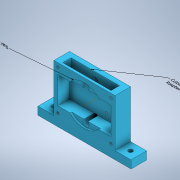
# Autodesk Inventor part: 2020PiZeroCameraLightRingMount
Saved by Autodesk Inventor 2020.2 (Build 242310000, 310)
## iProperties
Created: 2019-10-10
Part Number: 2020PiZeroCameraLightRingMount
Material: PC/ABS Plastic
Document SubType Name: Modeling
Designer: steele
Density: 0.357273 g/cm^3
Appearance: Turquoise
Author: steele
Autodesk Inventor part; units mm, degrees
ref_plane "YZ Plane" through (0, 0, 0) normal (1, 0, 0) x (0, 1, 0)
ref_plane "XZ Plane" through (0, 0, 0) normal (0, 1, 0) x (-1, 0, 0)
ref_plane "XY Plane" through (0, 0, 0) normal (0, 0, 1) x (1, 0, 0)
sketch "Sketch1" plane through (0, 0, 0) normal (0, 0, 1) x (1, 0, 0)
  line L0 (-48.5775, -37.85) -> (48.5775, -37.85)
  line L1 (48.5775, -37.85) -> (48.5775, 37.85)
  line L2 (48.5775, 37.85) -> (-48.5775, 37.85)
  line L3 (-48.5775, 37.85) -> (-48.5775, -37.85)
  line L4 (-48.5775, -37.85) -> (48.5775, 37.85) construction
  line L5 (48.5775, -37.85) -> (-48.5775, 37.85) construction
  point P0 (0, 0)
  dimension "majorPartWidth" = 97.155
  dimension "majorPartHeight" = 75.7
  constraints: 12 end point, 2 midpoint, 2 parallel, 1 horizontal, 1 perpendicular
  measures "majorPartWidth" distance of L0.start L0.end
  measures "majorPartHeight" distance of L1.end L0.end
extrude "Extrusion1" add sketch "Sketch1" against normal blind 24.725
sketch "Sketch2" plane through (0, 0, 0) normal (0, 0, 1) x (1, 0, 0)
  line L0 (-42.2275, -21.59) -> (42.2275, -21.59)
  line L1 (42.2275, -21.59) -> (42.2275, 21.59)
  line L2 (42.2275, 21.59) -> (-42.2275, 21.59)
  line L3 (-42.2275, 21.59) -> (-42.2275, -21.59)
  line L4 (-42.2275, -21.59) -> (42.2275, 21.59) construction
  line L5 (42.2275, -21.59) -> (-42.2275, 21.59) construction
  point P0 (0, 0)
  dimension "holeForPiCaseWidth" = 84.455
  dimension "holeForPiCaseHeight" = 43.18
  constraints: 12 end point, 2 midpoint, 2 parallel, 1 horizontal, 1 perpendicular
  measures "holeForPiCaseWidth" distance of L0.start L0.end
  measures "holeForPiCaseHeight" distance of L1.end L0.end
extrude "Extrusion2" cut sketch "Sketch2" against normal blind 18.375
sketch "Sketch3" plane through (0, 0, 0) normal (0, 0, 1) x (1, 0, 0)
  circle A0 centre (0, 0) radius 31.5
  circle A1 centre (0, 0) radius 18.5
  dimension "lightRingHoleExteriorDiam" = 63
  dimension "lightRingHoleInteriorDiam" = 37
  constraints: 2 centre point, 2 coincident
  measures "lightRingHoleExteriorDiam" diameter of A0
  measures "lightRingHoleInteriorDiam" diameter of A1
extrude "Extrusion3" cut sketch "Sketch3" against normal blind 2.5
sketch "Sketch4" plane through (0, 0, -2.5) normal (0, 0, 1) x (1, 0, 0)
  circle A0 centre (0, 0) radius 25.4466 construction
  circle A1 centre (0, 25.4466) radius 5
  circle A2 centre (0, -25.4466) radius 5
  dimension "holeForLightRingWires" = 10
  dimension "d13" = 10
  constraints: 3 centre point, 2 point on circle, 1 coincident
  measures "holeForLightRingWires" diameter of A1
  measures "d13" diameter of A2
extrude "Extrusion4" cut sketch "Sketch4" against normal through all
sketch "Sketch6" plane through (-48.5775, -37.85, 0) normal (0, -1, 0) x (1, 0, 0)
  line L0 (0, -24.725) -> (97.155, -24.725) projected
  line L1 (0, -24.725) -> (97.155, -24.725)
  line L2 (97.155, -24.725) -> (97.155, 0)
  line L3 (97.155, 0) -> (0, 0)
  line L4 (0, 0) -> (0, -24.725)
  point P0 (48.5775, 0)
  dimension "baseWidth" = 97.155
  dimension "baseDepth" = 24.725
  constraints: 8 end point, 2 parallel, 1 horizontal, 1 perpendicular
  measures "baseWidth" distance of L2.end L3.end
  measures "baseDepth" distance of L1.end L2.end
extrude "Extrusion6" add sketch "Sketch6" along normal blind 12.7
sketch "Sketch7" plane through (-48.5775, 37.85, 0) normal (0, 1, 0) x (1, 0, 0)
  line L0 (97.155, 0) -> (0, 0) construction
  line L1 (0, 0) -> (0, 24.725) construction
  line L2 (10.16, 3.77) -> (86.995, 3.77)
  line L3 (86.995, 3.77) -> (86.995, 17.105)
  line L4 (86.995, 17.105) -> (10.16, 17.105)
  line L5 (10.16, 17.105) -> (10.16, 3.77)
  line L6 (10.16, 3.77) -> (86.995, 17.105) construction
  line L7 (86.995, 3.77) -> (10.16, 17.105) construction
  line L8 (45.3952, 18.375) -> (45.3952, 2.5) projected
  point P0 (48.5775, 0)
  point P1 (48.5775, 10.4375)
  dimension "y" = 10.4375
  dimension "Y" = 48.5775
  dimension "piWireDepth" = 13.335
  dimension "piWireWidth" = 76.835
  constraints: 12 end point, 2 midpoint, 2 parallel, 2 perpendicular
  measures "y" distance from line of point (48.577, 10.438) L0
  measures "Y" distance from line of point (48.577, 10.438) L1
  measures "piWireDepth" distance of L4.end L2.start
  measures "piWireWidth" distance of L3.end L4.end
extrude "Extrusion7" cut sketch "Sketch7" against normal up to next
sketch "Sketch8" plane through (-48.5775, 37.85, -24.725) normal (-1, 0, 0) x (0, 0, 1)
  line L0 (24.725, -75.7) -> (24.725, 0) projected
  line L1 (24.725, -75.7) -> (28.535, -75.7)
  line L2 (28.535, -75.7) -> (28.535, -78.24)
  line L3 (28.535, -78.24) -> (24.725, -78.24)
  line L4 (24.725, -78.24) -> (24.725, -75.7)
  point P0 (24.725, -37.85)
  dimension "d30" = 3.81
  dimension "d31" = 2.54
  constraints: 8 end point, 2 parallel, 1 horizontal, 1 perpendicular
  measures "d30" distance of L2.end L3.end
  measures "d31" distance of L1.end L2.end
extrude "Extrusion8" cut sketch "Sketch8" against normal through all
sketch "Sketch9" plane through (0, 0, 0) normal (0, 0, 1) x (1, 0, 0)
  point P0 (-42.2275, 31.5)
  point P1 (42.2275, 31.5)
  point P2 (42.2275, -31.5)
  point P3 (-42.2275, -31.5)
hole "Hole1" at (-42.2275, 31.5, 0) at (42.2275, 31.5, 0) at (42.2275, -31.5, 0) at (-42.2275, -31.5, 0) direction (0, 0, -1) diameter 3.9624 depth 14.986 tip angle 120 thread size "10-32 UNF" class "2B" standard "ANSI Unified Screw Threads"
sketch "Sketch10" plane through (0, 0, -24.725) normal (0, 0, -1) x (-1, 0, 0)
  point P0 (-39.0525, 23.7022)
  point P1 (-16.8275, 23.7022)
  point P2 (-16.8275, -11.2228)
  point P3 (-39.0525, -11.2228)
hole "Hole3" at (39.0525, 23.7022, -24.725) at (16.8275, 23.7022, -24.725) at (16.8275, -11.2228, -24.725) at (39.0525, -11.2228, -24.725) direction (0, 0, 1) diameter 3.9624 depth 11.9507 tip angle 120 thread size "10-32 UNF" class "2B" standard "ANSI Unified Screw Threads"
sketch "Sketch14" plane through (-48.5775, -50.55, 0) normal (0, -1, 0) x (1, 0, 0)
  circle A0 centre (-12.7, 0) radius 2.5527 construction
  circle A1 centre (109.855, 0) radius 2.5527 construction
  line L0 (-12.7, 0) -> (109.855, 0) construction
  spline S0 degree 2 poles (41.3517, -2.5421) (41.3517, -2.8899) (41.0697, -3.4498) (40.833, -3.6062) knots 0 0 0 1 2 2 2
  spline S1 degree 2 poles (40.833, -3.6062) (40.6395, -3.7277) (40.2422, -3.81) (39.9335, -3.81) knots 0 0 0 1 2 2 2
  line L1 (39.9335, -3.81) -> (39.3489, -3.81)
  line L2 (39.3489, -3.81) -> (39.3489, -1.27)
  line L3 (39.3489, -1.27) -> (39.9273, -1.27)
  spline S2 degree 2 poles (39.9273, -1.27) (40.2854, -1.27) (40.693, -1.377) (40.8371, -1.4717) knots 0 0 0 1 2 2 2
  spline S3 degree 2 poles (40.8371, -1.4717) (41.082, -1.6343) (41.3517, -2.1716) (41.3517, -2.5421) knots 0 0 0 1 2 2 2
  spline S4 degree 2 poles (40.9997, -2.5379) (40.9997, -2.2457) (40.8062, -1.8319) (40.6148, -1.7146) knots 0 0 0 1 2 2 2
  spline S5 degree 2 poles (40.6148, -1.7146) (40.4789, -1.6343) (40.1722, -1.5623) (39.9438, -1.5623) knots 0 0 0 1 2 2 2
  line L4 (39.9438, -1.5623) -> (39.6865, -1.5623)
  line L5 (39.6865, -1.5623) -> (39.6865, -3.5177)
  line L6 (39.6865, -3.5177) -> (39.9438, -3.5177)
  spline S6 degree 2 poles (39.9438, -3.5177) (40.1681, -3.5177) (40.5078, -3.4457) (40.6457, -3.3489) knots 0 0 0 1 2 2 2
  spline S7 degree 2 poles (40.6457, -3.3489) (40.8227, -3.2295) (40.9997, -2.8343) (40.9997, -2.5379) knots 0 0 0 1 2 2 2
  spline S8 degree 2 poles (42.5208, -3.8532) (42.0639, -3.8532) (41.5616, -3.3407) (41.5616, -2.8673) knots 0 0 0 1 2 2 2
  spline S9 degree 2 poles (41.5616, -2.8673) (41.5616, -2.4021) (42.0495, -1.8505) (42.4426, -1.8505) knots 0 0 0 1 2 2 2
  spline S10 degree 2 poles (42.4426, -1.8505) (42.6196, -1.8505) (42.8934, -1.9534) (42.9942, -2.0625) knots 0 0 0 1 2 2 2
  spline S11 degree 2 poles (42.9942, -2.0625) (43.0972, -2.1716) (43.2062, -2.4865) (43.2062, -2.715) knots 0 0 0 1 2 2 2
  line L7 (43.2062, -2.715) -> (43.2062, -2.8899)
  line L8 (43.2062, -2.8899) -> (41.8868, -2.8899)
  spline S12 degree 2 poles (41.8868, -2.8899) (41.8868, -3.2213) (42.2203, -3.5733) (42.5167, -3.5733) knots 0 0 0 1 2 2 2
  spline S13 degree 2 poles (42.5167, -3.5733) (42.6217, -3.5733) (42.8254, -3.5259) (42.9078, -3.4889) knots 0 0 0 1 2 2 2
  spline S14 degree 2 poles (42.9078, -3.4889) (42.9942, -3.4477) (43.1136, -3.3757) (43.1527, -3.3428) knots 0 0 0 1 2 2 2
  line L9 (43.1527, -3.3428) -> (43.1713, -3.3428)
  line L10 (43.1713, -3.3428) -> (43.1713, -3.6927)
  spline S15 degree 2 poles (43.1713, -3.6927) (43.1157, -3.7153) (42.9469, -3.7812) (42.881, -3.7997) knots 0 0 0 1 2 2 2
  spline S16 degree 2 poles (42.881, -3.7997) (42.7884, -3.8265) (42.6361, -3.8532) (42.5208, -3.8532) knots 0 0 0 1 2 2 2
  spline S17 degree 2 poles (42.8934, -2.645) (42.8893, -2.5153) (42.8357, -2.3259) (42.7843, -2.2621) knots 0 0 0 1 2 2 2
  spline S18 degree 2 poles (42.7843, -2.2621) (42.7287, -2.1901) (42.5537, -2.1139) (42.4241, -2.1139) knots 0 0 0 1 2 2 2
  spline S19 degree 2 poles (42.4241, -2.1139) (42.2965, -2.1139) (42.1174, -2.1901) (42.0433, -2.2642) knots 0 0 0 1 2 2 2
  spline S20 degree 2 poles (42.0433, -2.2642) (41.9712, -2.3403) (41.8971, -2.5235) (41.8868, -2.645) knots 0 0 0 1 2 2 2
  line L11 (41.8868, -2.645) -> (42.8934, -2.645)
  spline S21 degree 2 poles (44.046, -3.8553) (43.8546, -3.8553) (43.5232, -3.7524) (43.4141, -3.6947) knots 0 0 0 1 2 2 2
  line L12 (43.4141, -3.6947) -> (43.4141, -3.3345)
  line L13 (43.4141, -3.3345) -> (43.4306, -3.3345)
  spline S22 degree 2 poles (43.4306, -3.3345) (43.4718, -3.3675) (43.5829, -3.4457) (43.6755, -3.4889) knots 0 0 0 1 2 2 2
  spline S23 degree 2 poles (43.6755, -3.4889) (43.7558, -3.528) (43.9534, -3.5856) (44.0584, -3.5856) knots 0 0 0 1 2 2 2
  spline S24 degree 2 poles (44.0584, -3.5856) (44.1346, -3.5856) (44.3095, -3.5506) (44.3507, -3.5218) knots 0 0 0 1 2 2 2
  spline S25 degree 2 poles (44.3507, -3.5218) (44.4104, -3.4827) (44.4639, -3.3942) (44.4639, -3.3036) knots 0 0 0 1 2 2 2
  spline S26 degree 2 poles (44.4639, -3.3036) (44.4639, -3.1904) (44.3404, -3.0731) (44.1819, -3.034) knots 0 0 0 1 2 2 2
  spline S27 degree 2 poles (44.1819, -3.034) (44.1202, -3.0196) (43.9225, -2.9784) (43.8382, -2.9558) knots 0 0 0 1 2 2 2
  spline S28 degree 2 poles (43.8382, -2.9558) (43.62, -2.892) (43.4224, -2.6285) (43.4224, -2.4412) knots 0 0 0 1 2 2 2
  spline S29 degree 2 poles (43.4224, -2.4412) (43.4224, -2.1818) (43.8114, -1.8587) (44.1325, -1.8587) knots 0 0 0 1 2 2 2
  spline S30 degree 2 poles (44.1325, -1.8587) (44.291, -1.8587) (44.6121, -1.9369) (44.7212, -1.9966) knots 0 0 0 1 2 2 2
  line L14 (44.7212, -1.9966) -> (44.7212, -2.3403)
  line L15 (44.7212, -2.3403) -> (44.7047, -2.3403)
  spline S31 degree 2 poles (44.7047, -2.3403) (44.5812, -2.2415) (44.2807, -2.1283) (44.1263, -2.1283) knots 0 0 0 1 2 2 2
  spline S32 degree 2 poles (44.1263, -2.1283) (43.9678, -2.1283) (43.7496, -2.2621) (43.7496, -2.3959) knots 0 0 0 1 2 2 2
  spline S33 degree 2 poles (43.7496, -2.3959) (43.7496, -2.5174) (43.8793, -2.6347) (44.0234, -2.6717) knots 0 0 0 1 2 2 2
  spline S34 degree 2 poles (44.0234, -2.6717) (44.0934, -2.6903) (44.2704, -2.7273) (44.3672, -2.75) knots 0 0 0 1 2 2 2
  spline S35 degree 2 poles (44.3672, -2.75) (44.5771, -2.8035) (44.7912, -3.0484) (44.7912, -3.2604) knots 0 0 0 1 2 2 2
  spline S36 degree 2 poles (44.7912, -3.2604) (44.7912, -3.3839) (44.6944, -3.6021) (44.5997, -3.6824) knots 0 0 0 1 2 2 2
  spline S37 degree 2 poles (44.5997, -3.6824) (44.4989, -3.7668) (44.2416, -3.8553) (44.046, -3.8553) knots 0 0 0 1 2 2 2
  line L16 (45.4169, -3.81) -> (45.0958, -3.81)
  line L17 (45.0958, -3.81) -> (45.0958, -1.904)
  line L18 (45.0958, -1.904) -> (45.4169, -1.904)
  line L19 (45.4169, -1.904) -> (45.4169, -3.81)
  line L20 (45.4396, -1.587) -> (45.0752, -1.587)
  line L21 (45.0752, -1.587) -> (45.0752, -1.2535)
  line L22 (45.0752, -1.2535) -> (45.4396, -1.2535)
  line L23 (45.4396, -1.2535) -> (45.4396, -1.587)
  spline S38 degree 2 poles (45.9562, -4.1146) (45.9891, -4.129) (46.1147, -4.1743) (46.195, -4.1929) knots 0 0 0 1 2 2 2
  spline S39 degree 2 poles (46.195, -4.1929) (46.2835, -4.2155) (46.4337, -4.2423) (46.5222, -4.2423) knots 0 0 0 1 2 2 2
  spline S40 degree 2 poles (46.5222, -4.2423) (46.6704, -4.2423) (46.8763, -4.164) (46.9339, -4.0941) knots 0 0 0 1 2 2 2
  spline S41 degree 2 poles (46.9339, -4.0941) (46.9895, -4.0241) (47.0327, -3.8409) (47.0327, -3.7235) knots 0 0 0 1 2 2 2
  line L24 (47.0327, -3.7235) -> (47.0327, -3.5568)
  spline S42 degree 2 poles (47.0327, -3.5568) (46.903, -3.67) (46.654, -3.7771) (46.4667, -3.7771) knots 0 0 0 1 2 2 2
  spline S43 degree 2 poles (46.4667, -3.7771) (46.1414, -3.7771) (45.7565, -3.2934) (45.7565, -2.8385) knots 0 0 0 1 2 2 2
  spline S44 degree 2 poles (45.7565, -2.8385) (45.7565, -2.6018) (45.8903, -2.2354) (46.0015, -2.1057) knots 0 0 0 1 2 2 2
  spline S45 degree 2 poles (46.0015, -2.1057) (46.1085, -1.9842) (46.4029, -1.8505) (46.5593, -1.8505) knots 0 0 0 1 2 2 2
  spline S46 degree 2 poles (46.5593, -1.8505) (46.7075, -1.8505) (46.9236, -1.9204) (47.0327, -1.9842) knots 0 0 0 1 2 2 2
  line L25 (47.0327, -1.9842) -> (47.0512, -1.904)
  line L26 (47.0512, -1.904) -> (47.3538, -1.904)
  line L27 (47.3538, -1.904) -> (47.3538, -3.5918)
  spline S47 degree 2 poles (47.3538, -3.5918) (47.3538, -4.0776) (46.9319, -4.5304) (46.4975, -4.5304) knots 0 0 0 1 2 2 2
  spline S48 degree 2 poles (46.4975, -4.5304) (46.3576, -4.5304) (46.0653, -4.4851) (45.9397, -4.4481) knots 0 0 0 1 2 2 2
  line L28 (45.9397, -4.4481) -> (45.9397, -4.1146)
  line L29 (45.9397, -4.1146) -> (45.9562, -4.1146)
  line L30 (47.0327, -3.2934) -> (47.0327, -2.2457)
  spline S49 degree 2 poles (47.0327, -2.2457) (46.9133, -2.188) (46.7116, -2.1386) (46.6107, -2.1386) knots 0 0 0 1 2 2 2
  spline S50 degree 2 poles (46.6107, -2.1386) (46.3679, -2.1386) (46.0879, -2.4968) (46.0879, -2.8323) knots 0 0 0 1 2 2 2
  spline S51 degree 2 poles (46.0879, -2.8323) (46.0879, -3.1493) (46.2999, -3.4807) (46.5387, -3.4807) knots 0 0 0 1 2 2 2
  spline S52 degree 2 poles (46.5387, -3.4807) (46.6643, -3.4807) (46.9277, -3.3819) (47.0327, -3.2934) knots 0 0 0 1 2 2 2
  line L31 (49.3154, -3.81) -> (48.9943, -3.81)
  line L32 (48.9943, -3.81) -> (48.9943, -2.7232)
  spline S53 degree 2 poles (48.9943, -2.7232) (48.9943, -2.5915) (48.9696, -2.365) (48.9326, -2.2971) knots 0 0 0 1 2 2 2
  spline S54 degree 2 poles (48.9326, -2.2971) (48.8935, -2.2251) (48.7535, -2.1551) (48.6341, -2.1551) knots 0 0 0 1 2 2 2
  spline S55 degree 2 poles (48.6341, -2.1551) (48.5147, -2.1551) (48.2615, -2.2827) (48.1401, -2.3856) knots 0 0 0 1 2 2 2
  line L33 (48.1401, -2.3856) -> (48.1401, -3.81)
  line L34 (48.1401, -3.81) -> (47.819, -3.81)
  line L35 (47.819, -3.81) -> (47.819, -1.904)
  line L36 (47.819, -1.904) -> (48.1401, -1.904)
  line L37 (48.1401, -1.904) -> (48.1401, -2.116)
  spline S56 degree 2 poles (48.1401, -2.116) (48.2842, -1.9863) (48.5621, -1.8505) (48.7185, -1.8505) knots 0 0 0 1 2 2 2
  spline S57 degree 2 poles (48.7185, -1.8505) (48.9984, -1.8505) (49.3154, -2.221) (49.3154, -2.5729) knots 0 0 0 1 2 2 2
  line L38 (49.3154, -2.5729) -> (49.3154, -3.81)
  spline S58 degree 2 poles (50.5937, -3.8532) (50.1367, -3.8532) (49.6345, -3.3407) (49.6345, -2.8673) knots 0 0 0 1 2 2 2
  spline S59 degree 2 poles (49.6345, -2.8673) (49.6345, -2.4021) (50.1223, -1.8505) (50.5154, -1.8505) knots 0 0 0 1 2 2 2
  spline S60 degree 2 poles (50.5154, -1.8505) (50.6925, -1.8505) (50.9662, -1.9534) (51.0671, -2.0625) knots 0 0 0 1 2 2 2
  spline S61 degree 2 poles (51.0671, -2.0625) (51.17, -2.1716) (51.2791, -2.4865) (51.2791, -2.715) knots 0 0 0 1 2 2 2
  line L39 (51.2791, -2.715) -> (51.2791, -2.8899)
  line L40 (51.2791, -2.8899) -> (49.9597, -2.8899)
  spline S62 degree 2 poles (49.9597, -2.8899) (49.9597, -3.2213) (50.2931, -3.5733) (50.5895, -3.5733) knots 0 0 0 1 2 2 2
  spline S63 degree 2 poles (50.5895, -3.5733) (50.6945, -3.5733) (50.8983, -3.5259) (50.9806, -3.4889) knots 0 0 0 1 2 2 2
  spline S64 degree 2 poles (50.9806, -3.4889) (51.0671, -3.4477) (51.1865, -3.3757) (51.2256, -3.3428) knots 0 0 0 1 2 2 2
  line L41 (51.2256, -3.3428) -> (51.2441, -3.3428)
  line L42 (51.2441, -3.3428) -> (51.2441, -3.6927)
  spline S65 degree 2 poles (51.2441, -3.6927) (51.1885, -3.7153) (51.0197, -3.7812) (50.9539, -3.7997) knots 0 0 0 1 2 2 2
  spline S66 degree 2 poles (50.9539, -3.7997) (50.8612, -3.8265) (50.7089, -3.8532) (50.5937, -3.8532) knots 0 0 0 1 2 2 2
  spline S67 degree 2 poles (50.9662, -2.645) (50.9621, -2.5153) (50.9086, -2.3259) (50.8571, -2.2621) knots 0 0 0 1 2 2 2
  spline S68 degree 2 poles (50.8571, -2.2621) (50.8015, -2.1901) (50.6266, -2.1139) (50.4969, -2.1139) knots 0 0 0 1 2 2 2
  spline S69 degree 2 poles (50.4969, -2.1139) (50.3693, -2.1139) (50.1902, -2.1901) (50.1161, -2.2642) knots 0 0 0 1 2 2 2
  spline S70 degree 2 poles (50.1161, -2.2642) (50.0441, -2.3403) (49.97, -2.5235) (49.9597, -2.645) knots 0 0 0 1 2 2 2
  line L43 (49.9597, -2.645) -> (50.9662, -2.645)
  line L44 (53.0698, -3.81) -> (52.7487, -3.81)
  line L45 (52.7487, -3.81) -> (52.7487, -3.6165)
  spline S71 degree 2 poles (52.7487, -3.6165) (52.6746, -3.6783) (52.5655, -3.7606) (52.4914, -3.7956) knots 0 0 0 1 2 2 2
  spline S72 degree 2 poles (52.4914, -3.7956) (52.4235, -3.8285) (52.2774, -3.8635) (52.1806, -3.8635) knots 0 0 0 1 2 2 2
  spline S73 degree 2 poles (52.1806, -3.8635) (52.0242, -3.8635) (51.7607, -3.7338) (51.6681, -3.6083) knots 0 0 0 1 2 2 2
  spline S74 degree 2 poles (51.6681, -3.6083) (51.5755, -3.4827) (51.4726, -3.1122) (51.4726, -2.8714) knots 0 0 0 1 2 2 2
  spline S75 degree 2 poles (51.4726, -2.8714) (51.4726, -2.6203) (51.6022, -2.2539) (51.7154, -2.116) knots 0 0 0 1 2 2 2
  spline S76 degree 2 poles (51.7154, -2.116) (51.8204, -1.9925) (52.1148, -1.8505) (52.2774, -1.8505) knots 0 0 0 1 2 2 2
  spline S77 degree 2 poles (52.2774, -1.8505) (52.4194, -1.8505) (52.6314, -1.9143) (52.7487, -1.9801) knots 0 0 0 1 2 2 2
  line L46 (52.7487, -1.9801) -> (52.7487, -1.1568)
  line L47 (52.7487, -1.1568) -> (53.0698, -1.1568)
  line L48 (53.0698, -1.1568) -> (53.0698, -3.81)
  line L49 (52.7487, -3.3469) -> (52.7487, -2.2457)
  spline S78 degree 2 poles (52.7487, -2.2457) (52.6294, -2.188) (52.44, -2.1448) (52.3309, -2.1448) knots 0 0 0 1 2 2 2
  spline S79 degree 2 poles (52.3309, -2.1448) (52.0839, -2.1448) (51.804, -2.5153) (51.804, -2.8652) knots 0 0 0 1 2 2 2
  spline S80 degree 2 poles (51.804, -2.8652) (51.804, -3.2028) (52.018, -3.5589) (52.2547, -3.5589) knots 0 0 0 1 2 2 2
  spline S81 degree 2 poles (52.2547, -3.5589) (52.3803, -3.5589) (52.6355, -3.4436) (52.7487, -3.3469) knots 0 0 0 1 2 2 2
  spline S82 degree 2 poles (56.2232, -2.8261) (56.2232, -3.2934) (55.7704, -3.8635) (55.4287, -3.8635) knots 0 0 0 1 2 2 2
  spline S83 degree 2 poles (55.4287, -3.8635) (55.2743, -3.8635) (55.0541, -3.7874) (54.9471, -3.7215) knots 0 0 0 1 2 2 2
  line L50 (54.9471, -3.7215) -> (54.9265, -3.81)
  line L51 (54.9265, -3.81) -> (54.626, -3.81)
  line L52 (54.626, -3.81) -> (54.626, -1.1568)
  line L53 (54.626, -1.1568) -> (54.9471, -1.1568)
  line L54 (54.9471, -1.1568) -> (54.9471, -2.1036)
  spline S84 degree 2 poles (54.9471, -2.1036) (55.0685, -1.9945) (55.3505, -1.8505) (55.5296, -1.8505) knots 0 0 0 1 2 2 2
  spline S85 degree 2 poles (55.5296, -1.8505) (55.8527, -1.8505) (56.2232, -2.3671) (56.2232, -2.8261) knots 0 0 0 1 2 2 2
  spline S86 degree 2 poles (55.8918, -2.8508) (55.8918, -2.5091) (55.6839, -2.1551) (55.4534, -2.1551) knots 0 0 0 1 2 2 2
  spline S87 degree 2 poles (55.4534, -2.1551) (55.3237, -2.1551) (55.0561, -2.2786) (54.9471, -2.3733) knots 0 0 0 1 2 2 2
  line L55 (54.9471, -2.3733) -> (54.9471, -3.4663)
  spline S88 degree 2 poles (54.9471, -3.4663) (55.0685, -3.5259) (55.2558, -3.5753) (55.367, -3.5753) knots 0 0 0 1 2 2 2
  spline S89 degree 2 poles (55.367, -3.5753) (55.6119, -3.5753) (55.8918, -3.2275) (55.8918, -2.8508) knots 0 0 0 1 2 2 2
  line L56 (58.0531, -1.904) -> (57.028, -4.5119)
  line L57 (57.028, -4.5119) -> (56.6843, -4.5119)
  line L58 (56.6843, -4.5119) -> (57.026, -3.7174)
  line L59 (57.026, -3.7174) -> (56.3344, -1.904)
  line L60 (56.3344, -1.904) -> (56.6802, -1.904)
  line L61 (56.6802, -1.904) -> (57.2009, -3.316)
  line L62 (57.2009, -3.316) -> (57.7196, -1.904)
  line L63 (57.7196, -1.904) -> (58.0531, -1.904)
  line L64 (42.5445, -8.0641) -> (42.1061, -8.0641)
  line L65 (42.1061, -8.0641) -> (41.3033, -7.0535)
  line L66 (41.3033, -7.0535) -> (40.9163, -7.0535)
  line L67 (40.9163, -7.0535) -> (40.9163, -8.0641)
  line L68 (40.9163, -8.0641) -> (40.5788, -8.0641)
  line L69 (40.5788, -8.0641) -> (40.5788, -5.5241)
  line L70 (40.5788, -5.5241) -> (41.2333, -5.5241)
  spline S90 degree 2 poles (41.2333, -5.5241) (41.4515, -5.5241) (41.7458, -5.5715) (41.8796, -5.6579) knots 0 0 0 1 2 2 2
  spline S91 degree 2 poles (41.8796, -5.6579) (42.0134, -5.7444) (42.1678, -6.014) (42.1678, -6.2137) knots 0 0 0 1 2 2 2
  spline S92 degree 2 poles (42.1678, -6.2137) (42.1678, -6.4916) (41.8838, -6.8682) (41.6409, -6.9588) knots 0 0 0 1 2 2 2
  line L71 (41.6409, -6.9588) -> (42.5445, -8.0641)
  spline S93 degree 2 poles (41.8158, -6.2404) (41.8158, -6.1293) (41.7376, -5.9585) (41.6553, -5.9029) knots 0 0 0 1 2 2 2
  spline S94 degree 2 poles (41.6553, -5.9029) (41.5832, -5.8555) (41.3918, -5.8164) (41.2518, -5.8164) knots 0 0 0 1 2 2 2
  line L72 (41.2518, -5.8164) -> (40.9163, -5.8164)
  line L73 (40.9163, -5.8164) -> (40.9163, -6.7715)
  line L74 (40.9163, -6.7715) -> (41.2127, -6.7715)
  spline S95 degree 2 poles (41.2127, -6.7715) (41.3589, -6.7715) (41.5915, -6.72) (41.6717, -6.6398) knots 0 0 0 1 2 2 2
  spline S96 degree 2 poles (41.6717, -6.6398) (41.7458, -6.5698) (41.8158, -6.3722) (41.8158, -6.2404) knots 0 0 0 1 2 2 2
  spline S97 degree 2 poles (44.2879, -7.1111) (44.2879, -7.5928) (43.8248, -8.1177) (43.4378, -8.1177) knots 0 0 0 1 2 2 2
  spline S98 degree 2 poles (43.4378, -8.1177) (43.0405, -8.1177) (42.5857, -7.5763) (42.5857, -7.1111) knots 0 0 0 1 2 2 2
  spline S99 degree 2 poles (42.5857, -7.1111) (42.5857, -6.6336) (43.055, -6.1046) (43.4378, -6.1046) knots 0 0 0 1 2 2 2
  spline S100 degree 2 poles (43.4378, -6.1046) (43.8248, -6.1046) (44.2879, -6.6315) (44.2879, -7.1111) knots 0 0 0 1 2 2 2
  spline S101 degree 2 poles (43.9565, -7.1111) (43.9565, -6.7406) (43.6869, -6.3804) (43.4378, -6.3804) knots 0 0 0 1 2 2 2
  spline S102 degree 2 poles (43.4378, -6.3804) (43.1887, -6.3804) (42.917, -6.7406) (42.917, -7.1111) knots 0 0 0 1 2 2 2
  spline S103 degree 2 poles (42.917, -7.1111) (42.917, -7.4713) (43.1887, -7.8418) (43.4378, -7.8418) knots 0 0 0 1 2 2 2
  spline S104 degree 2 poles (43.4378, -7.8418) (43.6848, -7.8418) (43.9565, -7.4775) (43.9565, -7.1111) knots 0 0 0 1 2 2 2
  spline S105 degree 2 poles (46.2145, -7.0803) (46.2145, -7.5475) (45.7617, -8.1177) (45.42, -8.1177) knots 0 0 0 1 2 2 2
  spline S106 degree 2 poles (45.42, -8.1177) (45.2656, -8.1177) (45.0454, -8.0415) (44.9383, -7.9756) knots 0 0 0 1 2 2 2
  line L75 (44.9383, -7.9756) -> (44.9178, -8.0641)
  line L76 (44.9178, -8.0641) -> (44.6172, -8.0641)
  line L77 (44.6172, -8.0641) -> (44.6172, -5.4109)
  line L78 (44.6172, -5.4109) -> (44.9383, -5.4109)
  line L79 (44.9383, -5.4109) -> (44.9383, -6.3578)
  spline S107 degree 2 poles (44.9383, -6.3578) (45.0598, -6.2487) (45.3418, -6.1046) (45.5209, -6.1046) knots 0 0 0 1 2 2 2
  spline S108 degree 2 poles (45.5209, -6.1046) (45.844, -6.1046) (46.2145, -6.6212) (46.2145, -7.0803) knots 0 0 0 1 2 2 2
  spline S109 degree 2 poles (45.8831, -7.105) (45.8831, -6.7633) (45.6752, -6.4092) (45.4447, -6.4092) knots 0 0 0 1 2 2 2
  spline S110 degree 2 poles (45.4447, -6.4092) (45.315, -6.4092) (45.0474, -6.5327) (44.9383, -6.6274) knots 0 0 0 1 2 2 2
  line L80 (44.9383, -6.6274) -> (44.9383, -7.7204)
  spline S111 degree 2 poles (44.9383, -7.7204) (45.0598, -7.7801) (45.2471, -7.8295) (45.3582, -7.8295) knots 0 0 0 1 2 2 2
  spline S112 degree 2 poles (45.3582, -7.8295) (45.6032, -7.8295) (45.8831, -7.4816) (45.8831, -7.105) knots 0 0 0 1 2 2 2
  spline S113 degree 2 poles (48.3717, -8.1094) (48.0958, -8.1094) (47.7089, -7.9942) (47.538, -7.9118) knots 0 0 0 1 2 2 2
  line L81 (47.538, -7.9118) -> (47.538, -7.4878)
  line L82 (47.538, -7.4878) -> (47.5627, -7.4878)
  spline S114 degree 2 poles (47.5627, -7.4878) (47.7295, -7.6442) (48.1514, -7.8171) (48.347, -7.8171) knots 0 0 0 1 2 2 2
  spline S115 degree 2 poles (48.347, -7.8171) (48.6269, -7.8171) (48.913, -7.5845) (48.913, -7.3931) knots 0 0 0 1 2 2 2
  spline S116 degree 2 poles (48.913, -7.3931) (48.913, -7.2408) (48.7628, -7.0514) (48.6001, -7.0041) knots 0 0 0 1 2 2 2
  spline S117 degree 2 poles (48.6001, -7.0041) (48.4828, -6.9712) (48.2873, -6.9259) (48.1411, -6.8888) knots 0 0 0 1 2 2 2
  spline S118 degree 2 poles (48.1411, -6.8888) (48.0094, -6.8538) (47.8015, -6.7489) (47.7212, -6.6645) knots 0 0 0 1 2 2 2
  spline S119 degree 2 poles (47.7212, -6.6645) (47.643, -6.5801) (47.5566, -6.3537) (47.5566, -6.2055) knots 0 0 0 1 2 2 2
  spline S120 degree 2 poles (47.5566, -6.2055) (47.5566, -5.8967) (48.0382, -5.4789) (48.4108, -5.4789) knots 0 0 0 1 2 2 2
  spline S121 degree 2 poles (48.4108, -5.4789) (48.6248, -5.4789) (49.0036, -5.5633) (49.1662, -5.6435) knots 0 0 0 1 2 2 2
  line L83 (49.1662, -5.6435) -> (49.1662, -6.047)
  line L84 (49.1662, -6.047) -> (49.1415, -6.047)
  spline S122 degree 2 poles (49.1415, -6.047) (49.02, -5.9358) (48.6413, -5.7711) (48.4334, -5.7711) knots 0 0 0 1 2 2 2
  spline S123 degree 2 poles (48.4334, -5.7711) (48.1988, -5.7711) (47.9085, -5.9914) (47.9085, -6.1705) knots 0 0 0 1 2 2 2
  spline S124 degree 2 poles (47.9085, -6.1705) (47.9085, -6.331) (48.0794, -6.5224) (48.2399, -6.5657) knots 0 0 0 1 2 2 2
  spline S125 degree 2 poles (48.2399, -6.5657) (48.347, -6.5945) (48.6578, -6.6686) (48.7607, -6.6995) knots 0 0 0 1 2 2 2
  spline S126 degree 2 poles (48.7607, -6.6995) (49.0221, -6.7797) (49.265, -7.1029) (49.265, -7.3396) knots 0 0 0 1 2 2 2
  spline S127 degree 2 poles (49.265, -7.3396) (49.265, -7.4899) (49.1435, -7.778) (49.0345, -7.8789) knots 0 0 0 1 2 2 2
  spline S128 degree 2 poles (49.0345, -7.8789) (48.913, -7.99) (48.6043, -8.1094) (48.3717, -8.1094) knots 0 0 0 1 2 2 2
  spline S129 degree 2 poles (50.1604, -8.1012) (49.899, -8.1012) (49.6046, -7.8027) (49.6046, -7.4796) knots 0 0 0 1 2 2 2
  line L85 (49.6046, -7.4796) -> (49.6046, -6.4236)
  line L86 (49.6046, -6.4236) -> (49.3885, -6.4236)
  line L87 (49.3885, -6.4236) -> (49.3885, -6.1581)
  line L88 (49.3885, -6.1581) -> (49.6046, -6.1581)
  line L89 (49.6046, -6.1581) -> (49.6046, -5.6106)
  line L90 (49.6046, -5.6106) -> (49.9257, -5.6106)
  line L91 (49.9257, -5.6106) -> (49.9257, -6.1581)
  line L92 (49.9257, -6.1581) -> (50.5165, -6.1581)
  line L93 (50.5165, -6.1581) -> (50.5165, -6.4236)
  line L94 (50.5165, -6.4236) -> (49.9257, -6.4236)
  line L95 (49.9257, -6.4236) -> (49.9257, -7.3314)
  spline S130 degree 2 poles (49.9257, -7.3314) (49.9257, -7.4755) (49.936, -7.6339) (49.971, -7.7019) knots 0 0 0 1 2 2 2
  spline S131 degree 2 poles (49.971, -7.7019) (49.9998, -7.7616) (50.1295, -7.8213) (50.2406, -7.8213) knots 0 0 0 1 2 2 2
  spline S132 degree 2 poles (50.2406, -7.8213) (50.3189, -7.8213) (50.465, -7.7739) (50.4979, -7.7595) knots 0 0 0 1 2 2 2
  line L96 (50.4979, -7.7595) -> (50.5165, -7.7595)
  line L97 (50.5165, -7.7595) -> (50.5165, -8.0477)
  spline S133 degree 2 poles (50.5165, -8.0477) (50.4259, -8.0724) (50.2406, -8.1012) (50.1604, -8.1012) knots 0 0 0 1 2 2 2
  spline S134 degree 2 poles (51.5806, -8.1074) (51.1237, -8.1074) (50.6214, -7.5948) (50.6214, -7.1214) knots 0 0 0 1 2 2 2
  spline S135 degree 2 poles (50.6214, -7.1214) (50.6214, -6.6562) (51.1093, -6.1046) (51.5024, -6.1046) knots 0 0 0 1 2 2 2
  spline S136 degree 2 poles (51.5024, -6.1046) (51.6794, -6.1046) (51.9532, -6.2075) (52.054, -6.3166) knots 0 0 0 1 2 2 2
  spline S137 degree 2 poles (52.054, -6.3166) (52.157, -6.4257) (52.2661, -6.7406) (52.2661, -6.9691) knots 0 0 0 1 2 2 2
  line L98 (52.2661, -6.9691) -> (52.2661, -7.1441)
  line L99 (52.2661, -7.1441) -> (50.9467, -7.1441)
  spline S138 degree 2 poles (50.9467, -7.1441) (50.9467, -7.4755) (51.2801, -7.8274) (51.5765, -7.8274) knots 0 0 0 1 2 2 2
  spline S139 degree 2 poles (51.5765, -7.8274) (51.6815, -7.8274) (51.8853, -7.7801) (51.9676, -7.743) knots 0 0 0 1 2 2 2
  spline S140 degree 2 poles (51.9676, -7.743) (52.054, -7.7019) (52.1734, -7.6298) (52.2125, -7.5969) knots 0 0 0 1 2 2 2
  line L100 (52.2125, -7.5969) -> (52.2311, -7.5969)
  line L101 (52.2311, -7.5969) -> (52.2311, -7.9468)
  spline S141 degree 2 poles (52.2311, -7.9468) (52.1755, -7.9695) (52.0067, -8.0353) (51.9408, -8.0539) knots 0 0 0 1 2 2 2
  spline S142 degree 2 poles (51.9408, -8.0539) (51.8482, -8.0806) (51.6959, -8.1074) (51.5806, -8.1074) knots 0 0 0 1 2 2 2
  spline S143 degree 2 poles (51.9532, -6.8991) (51.9491, -6.7694) (51.8956, -6.5801) (51.8441, -6.5163) knots 0 0 0 1 2 2 2
  spline S144 degree 2 poles (51.8441, -6.5163) (51.7885, -6.4442) (51.6136, -6.3681) (51.4839, -6.3681) knots 0 0 0 1 2 2 2
  spline S145 degree 2 poles (51.4839, -6.3681) (51.3563, -6.3681) (51.1772, -6.4442) (51.1031, -6.5183) knots 0 0 0 1 2 2 2
  spline S146 degree 2 poles (51.1031, -6.5183) (51.031, -6.5945) (50.9569, -6.7777) (50.9467, -6.8991) knots 0 0 0 1 2 2 2
  line L102 (50.9467, -6.8991) -> (51.9532, -6.8991)
  spline S147 degree 2 poles (53.4187, -8.1074) (52.9618, -8.1074) (52.4595, -7.5948) (52.4595, -7.1214) knots 0 0 0 1 2 2 2
  spline S148 degree 2 poles (52.4595, -7.1214) (52.4595, -6.6562) (52.9474, -6.1046) (53.3405, -6.1046) knots 0 0 0 1 2 2 2
  spline S149 degree 2 poles (53.3405, -6.1046) (53.5175, -6.1046) (53.7913, -6.2075) (53.8922, -6.3166) knots 0 0 0 1 2 2 2
  spline S150 degree 2 poles (53.8922, -6.3166) (53.9951, -6.4257) (54.1042, -6.7406) (54.1042, -6.9691) knots 0 0 0 1 2 2 2
  line L103 (54.1042, -6.9691) -> (54.1042, -7.1441)
  line L104 (54.1042, -7.1441) -> (52.7848, -7.1441)
  spline S151 degree 2 poles (52.7848, -7.1441) (52.7848, -7.4755) (53.1182, -7.8274) (53.4146, -7.8274) knots 0 0 0 1 2 2 2
  spline S152 degree 2 poles (53.4146, -7.8274) (53.5196, -7.8274) (53.7234, -7.7801) (53.8057, -7.743) knots 0 0 0 1 2 2 2
  spline S153 degree 2 poles (53.8057, -7.743) (53.8922, -7.7019) (54.0115, -7.6298) (54.0506, -7.5969) knots 0 0 0 1 2 2 2
  line L105 (54.0506, -7.5969) -> (54.0692, -7.5969)
  line L106 (54.0692, -7.5969) -> (54.0692, -7.9468)
  spline S154 degree 2 poles (54.0692, -7.9468) (54.0136, -7.9695) (53.8448, -8.0353) (53.7789, -8.0539) knots 0 0 0 1 2 2 2
  spline S155 degree 2 poles (53.7789, -8.0539) (53.6863, -8.0806) (53.534, -8.1074) (53.4187, -8.1074) knots 0 0 0 1 2 2 2
  spline S156 degree 2 poles (53.7913, -6.8991) (53.7872, -6.7694) (53.7337, -6.5801) (53.6822, -6.5163) knots 0 0 0 1 2 2 2
  spline S157 degree 2 poles (53.6822, -6.5163) (53.6266, -6.4442) (53.4517, -6.3681) (53.322, -6.3681) knots 0 0 0 1 2 2 2
  spline S158 degree 2 poles (53.322, -6.3681) (53.1944, -6.3681) (53.0153, -6.4442) (52.9412, -6.5183) knots 0 0 0 1 2 2 2
  spline S159 degree 2 poles (52.9412, -6.5183) (52.8692, -6.5945) (52.7951, -6.7777) (52.7848, -6.8991) knots 0 0 0 1 2 2 2
  line L107 (52.7848, -6.8991) -> (53.7913, -6.8991)
  line L108 (54.7567, -8.0641) -> (54.4356, -8.0641)
  line L109 (54.4356, -8.0641) -> (54.4356, -5.4109)
  line L110 (54.4356, -5.4109) -> (54.7567, -5.4109)
  line L111 (54.7567, -5.4109) -> (54.7567, -8.0641)
  spline S160 degree 2 poles (56.0555, -8.1074) (55.5985, -8.1074) (55.0963, -7.5948) (55.0963, -7.1214) knots 0 0 0 1 2 2 2
  spline S161 degree 2 poles (55.0963, -7.1214) (55.0963, -6.6562) (55.5841, -6.1046) (55.9773, -6.1046) knots 0 0 0 1 2 2 2
  spline S162 degree 2 poles (55.9773, -6.1046) (56.1543, -6.1046) (56.428, -6.2075) (56.5289, -6.3166) knots 0 0 0 1 2 2 2
  spline S163 degree 2 poles (56.5289, -6.3166) (56.6318, -6.4257) (56.7409, -6.7406) (56.7409, -6.9691) knots 0 0 0 1 2 2 2
  line L112 (56.7409, -6.9691) -> (56.7409, -7.1441)
  line L113 (56.7409, -7.1441) -> (55.4215, -7.1441)
  spline S164 degree 2 poles (55.4215, -7.1441) (55.4215, -7.4755) (55.755, -7.8274) (56.0514, -7.8274) knots 0 0 0 1 2 2 2
  spline S165 degree 2 poles (56.0514, -7.8274) (56.1563, -7.8274) (56.3601, -7.7801) (56.4424, -7.743) knots 0 0 0 1 2 2 2
  spline S166 degree 2 poles (56.4424, -7.743) (56.5289, -7.7019) (56.6483, -7.6298) (56.6874, -7.5969) knots 0 0 0 1 2 2 2
  line L114 (56.6874, -7.5969) -> (56.7059, -7.5969)
  line L115 (56.7059, -7.5969) -> (56.7059, -7.9468)
  spline S167 degree 2 poles (56.7059, -7.9468) (56.6503, -7.9695) (56.4816, -8.0353) (56.4157, -8.0539) knots 0 0 0 1 2 2 2
  spline S168 degree 2 poles (56.4157, -8.0539) (56.3231, -8.0806) (56.1707, -8.1074) (56.0555, -8.1074) knots 0 0 0 1 2 2 2
  spline S169 degree 2 poles (56.428, -6.8991) (56.4239, -6.7694) (56.3704, -6.5801) (56.3189, -6.5163) knots 0 0 0 1 2 2 2
  spline S170 degree 2 poles (56.3189, -6.5163) (56.2634, -6.4442) (56.0884, -6.3681) (55.9587, -6.3681) knots 0 0 0 1 2 2 2
  spline S171 degree 2 poles (55.9587, -6.3681) (55.8311, -6.3681) (55.652, -6.4442) (55.5779, -6.5183) knots 0 0 0 1 2 2 2
  spline S172 degree 2 poles (55.5779, -6.5183) (55.5059, -6.5945) (55.4318, -6.7777) (55.4215, -6.8991) knots 0 0 0 1 2 2 2
  line L116 (55.4215, -6.8991) -> (56.428, -6.8991)
  line L117 (47.7284, -9.7186) -> (46.8536, -12.2586)
  line L118 (46.8536, -12.2586) -> (46.4893, -12.2586)
  line L119 (46.4893, -12.2586) -> (45.6145, -9.7186)
  line L120 (45.6145, -9.7186) -> (45.9768, -9.7186)
  line L121 (45.9768, -9.7186) -> (46.6807, -11.8284)
  line L122 (46.6807, -11.8284) -> (47.3847, -9.7186)
  line L123 (47.3847, -9.7186) -> (47.7284, -9.7186)
  spline S173 degree 2 poles (49.5089, -10.9886) (49.5089, -11.672) (49.1116, -12.3121) (48.6979, -12.3121) knots 0 0 0 1 2 2 2
  spline S174 degree 2 poles (48.6979, -12.3121) (48.278, -12.3121) (47.8849, -11.6596) (47.8849, -10.9907) knots 0 0 0 1 2 2 2
  spline S175 degree 2 poles (47.8849, -10.9907) (47.8849, -10.3032) (48.2821, -9.6671) (48.6979, -9.6671) knots 0 0 0 1 2 2 2
  spline S176 degree 2 poles (48.6979, -9.6671) (49.1158, -9.6671) (49.5089, -10.3258) (49.5089, -10.9886) knots 0 0 0 1 2 2 2
  spline S177 degree 2 poles (49.0725, -11.7625) (49.1219, -11.637) (49.1631, -11.25) (49.1631, -10.9886) knots 0 0 0 1 2 2 2
  spline S178 degree 2 poles (49.1631, -10.9886) (49.1631, -10.7272) (49.1219, -10.3423) (49.0705, -10.2126) knots 0 0 0 1 2 2 2
  spline S179 degree 2 poles (49.0705, -10.2126) (49.019, -10.0829) (48.8399, -9.9491) (48.6979, -9.9491) knots 0 0 0 1 2 2 2
  spline S180 degree 2 poles (48.6979, -9.9491) (48.5559, -9.9491) (48.3727, -10.0829) (48.3192, -10.2167) knots 0 0 0 1 2 2 2
  spline S181 degree 2 poles (48.3192, -10.2167) (48.2677, -10.3464) (48.2307, -10.7416) (48.2307, -10.9907) knots 0 0 0 1 2 2 2
  spline S182 degree 2 poles (48.2307, -10.9907) (48.2307, -11.2582) (48.2636, -11.6164) (48.3171, -11.7564) knots 0 0 0 1 2 2 2
  spline S183 degree 2 poles (48.3171, -11.7564) (48.3665, -11.8881) (48.5497, -12.0301) (48.6979, -12.0301) knots 0 0 0 1 2 2 2
  spline S184 degree 2 poles (48.6979, -12.0301) (48.8379, -12.0301) (49.0211, -11.8963) (49.0725, -11.7625) knots 0 0 0 1 2 2 2
  spline S185 degree 2 poles (50.5196, -9.9594) (50.4269, -9.9594) (50.2437, -10.0047) (50.1552, -10.0397) knots 0 0 0 1 2 2 2
  spline S186 degree 2 poles (50.1552, -10.0397) (50.0729, -10.0747) (49.9514, -10.1488) (49.9041, -10.1817) knots 0 0 0 1 2 2 2
  line L124 (49.9041, -10.1817) -> (49.8835, -10.1817)
  line L125 (49.8835, -10.1817) -> (49.8835, -9.8215)
  spline S187 degree 2 poles (49.8835, -9.8215) (49.9947, -9.7618) (50.3755, -9.6651) (50.5463, -9.6651) knots 0 0 0 1 2 2 2
  spline S188 degree 2 poles (50.5463, -9.6651) (50.7192, -9.6651) (50.9765, -9.7351) (51.0815, -9.8092) knots 0 0 0 1 2 2 2
  spline S189 degree 2 poles (51.0815, -9.8092) (51.1926, -9.8894) (51.3079, -10.122) (51.3079, -10.2785) knots 0 0 0 1 2 2 2
  spline S190 degree 2 poles (51.3079, -10.2785) (51.3079, -10.4884) (51.0321, -10.8054) (50.8386, -10.8466) knots 0 0 0 1 2 2 2
  line L126 (50.8386, -10.8466) -> (50.8386, -10.8713)
  spline S191 degree 2 poles (50.8386, -10.8713) (50.9189, -10.8877) (51.1021, -10.9618) (51.1803, -11.0359) knots 0 0 0 1 2 2 2
  spline S192 degree 2 poles (51.1803, -11.0359) (51.2585, -11.108) (51.3573, -11.3385) (51.3573, -11.5052) knots 0 0 0 1 2 2 2
  spline S193 degree 2 poles (51.3573, -11.5052) (51.3573, -11.6761) (51.24, -11.9663) (51.1329, -12.0775) knots 0 0 0 1 2 2 2
  spline S194 degree 2 poles (51.1329, -12.0775) (51.0218, -12.1927) (50.7069, -12.3121) (50.5072, -12.3121) knots 0 0 0 1 2 2 2
  spline S195 degree 2 poles (50.5072, -12.3121) (50.3158, -12.3121) (49.9412, -12.2195) (49.8135, -12.1557) knots 0 0 0 1 2 2 2
  line L127 (49.8135, -12.1557) -> (49.8135, -11.7955)
  line L128 (49.8135, -11.7955) -> (49.8382, -11.7955)
  spline S196 degree 2 poles (49.8382, -11.7955) (49.9453, -11.8737) (50.3075, -12.0178) (50.4866, -12.0178) knots 0 0 0 1 2 2 2
  spline S197 degree 2 poles (50.4866, -12.0178) (50.5916, -12.0178) (50.8015, -11.9519) (50.8715, -11.8757) knots 0 0 0 1 2 2 2
  spline S198 degree 2 poles (50.8715, -11.8757) (50.9395, -11.7996) (51.0115, -11.6185) (51.0115, -11.4805) knots 0 0 0 1 2 2 2
  spline S199 degree 2 poles (51.0115, -11.4805) (51.0115, -11.3426) (50.9312, -11.1636) (50.8592, -11.1121) knots 0 0 0 1 2 2 2
  spline S200 degree 2 poles (50.8592, -11.1121) (50.7871, -11.0606) (50.5916, -11.0215) (50.4763, -11.0215) knots 0 0 0 1 2 2 2
  line L129 (50.4763, -11.0215) -> (50.3322, -11.0215)
  line L130 (50.3322, -11.0215) -> (50.3322, -10.7395)
  line L131 (50.3322, -10.7395) -> (50.4454, -10.7395)
  spline S201 degree 2 poles (50.4454, -10.7395) (50.6739, -10.7395) (50.9621, -10.5214) (50.9621, -10.3135) knots 0 0 0 1 2 2 2
  spline S202 degree 2 poles (50.9621, -10.3135) (50.9621, -10.2167) (50.888, -10.0788) (50.8283, -10.0376) knots 0 0 0 1 2 2 2
  spline S203 degree 2 poles (50.8283, -10.0376) (50.7645, -9.9944) (50.6081, -9.9594) (50.5196, -9.9594) knots 0 0 0 1 2 2 2
  point P0 (48.5775, 0)
  constraints: 2 end point, 2 horizontal
extrude "Extrusion11" cut sketch "Sketch14" against normal blind 3.175
sketch "Sketch15" plane through (48.5775, 37.85, 0) normal (1, 0, 0) x (0, 0, -1)
  line L0 (24.725, 0) -> (24.725, -88.4) projected
  line L1 (0, -88.4) -> (24.725, -88.4)
  line L2 (24.725, -88.4) -> (24.725, -75.7)
  line L3 (24.725, -75.7) -> (0, -75.7)
  line L4 (0, -75.7) -> (0, -88.4)
  point P0 (0, -37.85)
  dimension "d68" = 12.7
  constraints: 8 end point, 2 parallel, 1 horizontal, 1 perpendicular, 1 point on line
  measures "d68" distance of L2.end L1.end
extrude "Extrusion12" add sketch "Sketch15" along normal blind 25.4
sketch "Sketch16" plane through (48.5775, -37.85, 0) normal (0, 1, 0) x (1, 0, 0)
  line L0 (0, 24.725) -> (25.4, 24.725) projected
  line L1 (0, 0) -> (0, 24.725) projected
  point P0 (-48.5775, 0)
  point P1 (12.7, 12.025)
  dimension "d78" = 12.7
  dimension "d79" = 12.7
  measures "d78" distance from line of point (12.7, 12.025) L0
  measures "d79" distance from line of point (12.7, 12.025) L1
hole "Hole6" at (61.2775, -37.85, -12.025) direction (0, -1, 0) diameter 6.7564 end through all
mirror "Mirror2" about plane through (0, 0, 0) normal (1, 0, 0) of "Extrusion12", "Hole6"
equation "\"majorPartWidth\" = holeForPiCaseWidth + 2 * minWallThickness"
equation "\"majorPartHeight\" = lightRingHoleExteriorDiam + 2 * minWallThickness"
equation "\"majorPartDepth\" = holeForPiCaseDepth + minWallThickness"
equation "\"holeForPiCaseWidth\" = piCaseWidth + 2 * caseGap"
equation "\"holeForPiCaseHeight\" = piCaseHeight + 2 * caseGap"
equation "\"holeForPiCaseDepth\" = PiCaseDepth + depthForLightRing"
equation "\"lightRingHoleExteriorDiam\" = lightRingExteriorDiam + lightRingEdgeSpacing"
equation "\"lightRingHoleInteriorDiam\" = lightRingInterorDiam - lightRingEdgeSpacing"
equation "\"d13\" = holeForLightRingWires"
equation "\"baseWidth\" = majorPartWidth"
equation "\"baseDepth\" = majorPartDepth"
equation "\"y\" = 0.5 * PiCaseDepth + depthForLightRing"
equation "\"Y\" = 0.5 * majorPartWidth"
equation "\"minWallThickness\" = 6.35"
equation "\"lightRingEdgeSpacing\" = 3"
equation "\"lightRingExteriorDiam\" = 60"
equation "\"lightRingInterorDiam\" = 40"
equation "\"caseGap\" = 2.54"
equation "\"piCaseWidth\" = 79.375"
equation "\"piCaseHeight\" = 38.1"
equation "\"PiCaseDepth\" = 15.875"
equation "\"depthForLightRing\" = 2.5"
body "Solid1"
